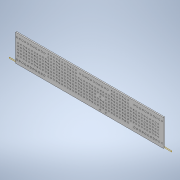
# Autodesk Inventor part: top_plate
Saved by Autodesk Inventor 2022 (Build 260153000, 153)
## iProperties
Created: 2021-07-14
Part Number: top_plate
Material: Generic
Document SubType Name: Modeling
Designer: gfellows
Density: 1 g/cm^3
Appearance: Default
Author: gfellows
Autodesk Inventor part; units mm, degrees
ref_plane "YZ Plane" through (0, 0, 0) normal (1, 0, 0) x (0, 1, 0)
ref_plane "XZ Plane" through (0, 0, 0) normal (0, 1, 0) x (-1, 0, 0)
ref_plane "XY Plane" through (0, 0, 0) normal (0, 0, 1) x (1, 0, 0)
ref_plane "Work Plane1" through (-368.7905, 0, 55) normal (0, 0, 1) x (1, 0, 0)
sketch "Sketch1" plane through (-368.7905, 0, 55) normal (0, 0, 1) x (1, 0, 0)
  line L0 (0, 0) -> (430.2, 0)
  line L1 (430.2, 0) -> (430.2, 78.35)
  line L2 (430.2, 78.35) -> (0, 78.35)
  line L3 (0, 78.35) -> (0, 0)
  circle A0 centre (262.5182, 6.225) radius 1.3525 projected
  line L4 (229.7522, 3.429) -> (229.7522, 41.021) projected
  line L5 (268.9952, 3.429) -> (229.7522, 3.429) projected
  line L6 (268.9952, 41.021) -> (268.9952, 3.429) projected
  line L7 (229.7522, 41.021) -> (268.9952, 41.021) projected
  circle A1 centre (262.5182, 6.225) radius 1.3525 projected
  circle A2 centre (246.5182, 6.225) radius 1.3525 projected
  circle A3 centre (262.5182, 38.225) radius 1.3525 projected
  circle A4 centre (246.5182, 38.225) radius 1.3525 projected
  circle A5 centre (-0.4541, 14.35) radius 1.65
  line L8 (0, 75.175) -> (0, 78.35) projected
  line L9 (0, 0) -> (430.2, 0) projected
  circle A6 centre (-0.4541, 22.35) radius 1.65
  circle A7 centre (-0.4541, 30.35) radius 1.65
  circle A8 centre (-0.4541, 38.35) radius 1.65
  circle A9 centre (-0.4541, 46.35) radius 1.65
  circle A10 centre (-0.4541, 54.35) radius 1.65
  circle A11 centre (-0.4541, 62.35) radius 1.65
  circle A12 centre (-0.4541, 70.35) radius 1.65
  circle A13 centre (7.5459, 14.35) radius 1.65
  circle A14 centre (7.5459, 22.35) radius 1.65
  circle A15 centre (7.5459, 30.35) radius 1.65
  circle A16 centre (7.5459, 38.35) radius 1.65
  circle A17 centre (7.5459, 46.35) radius 1.65
  circle A18 centre (7.5459, 54.35) radius 1.65
  circle A19 centre (7.5459, 62.35) radius 1.65
  circle A20 centre (7.5459, 70.35) radius 1.65
  circle A21 centre (15.5459, 14.35) radius 1.65
  circle A22 centre (15.5459, 22.35) radius 1.65
  circle A23 centre (15.5459, 30.35) radius 1.65
  circle A24 centre (15.5459, 38.35) radius 1.65
  circle A25 centre (15.5459, 46.35) radius 1.65
  circle A26 centre (15.5459, 54.35) radius 1.65
  circle A27 centre (15.5459, 62.35) radius 1.65
  circle A28 centre (15.5459, 70.35) radius 1.65
  circle A29 centre (23.5459, 14.35) radius 1.65
  circle A30 centre (23.5459, 22.35) radius 1.65
  circle A31 centre (23.5459, 30.35) radius 1.65
  circle A32 centre (23.5459, 38.35) radius 1.65
  circle A33 centre (23.5459, 46.35) radius 1.65
  circle A34 centre (23.5459, 54.35) radius 1.65
  circle A35 centre (23.5459, 62.35) radius 1.65
  circle A36 centre (23.5459, 70.35) radius 1.65
  circle A37 centre (31.5459, 14.35) radius 1.65
  circle A38 centre (31.5459, 22.35) radius 1.65
  circle A39 centre (31.5459, 30.35) radius 1.65
  circle A40 centre (31.5459, 38.35) radius 1.65
  circle A41 centre (31.5459, 46.35) radius 1.65
  circle A42 centre (31.5459, 54.35) radius 1.65
  circle A43 centre (31.5459, 62.35) radius 1.65
  circle A44 centre (31.5459, 70.35) radius 1.65
  circle A45 centre (39.5459, 14.35) radius 1.65
  circle A46 centre (39.5459, 22.35) radius 1.65
  circle A47 centre (39.5459, 30.35) radius 1.65
  circle A48 centre (39.5459, 38.35) radius 1.65
  circle A49 centre (39.5459, 46.35) radius 1.65
  circle A50 centre (39.5459, 54.35) radius 1.65
  circle A51 centre (39.5459, 62.35) radius 1.65
  circle A52 centre (39.5459, 70.35) radius 1.65
  circle A53 centre (47.5459, 14.35) radius 1.65
  circle A54 centre (47.5459, 22.35) radius 1.65
  circle A55 centre (47.5459, 30.35) radius 1.65
  circle A56 centre (47.5459, 38.35) radius 1.65
  circle A57 centre (47.5459, 46.35) radius 1.65
  circle A58 centre (47.5459, 54.35) radius 1.65
  circle A59 centre (47.5459, 62.35) radius 1.65
  circle A60 centre (47.5459, 70.35) radius 1.65
  circle A61 centre (55.5459, 14.35) radius 1.65
  circle A62 centre (55.5459, 22.35) radius 1.65
  circle A63 centre (55.5459, 30.35) radius 1.65
  circle A64 centre (55.5459, 38.35) radius 1.65
  circle A65 centre (55.5459, 46.35) radius 1.65
  circle A66 centre (55.5459, 54.35) radius 1.65
  circle A67 centre (55.5459, 62.35) radius 1.65
  circle A68 centre (55.5459, 70.35) radius 1.65
  circle A69 centre (63.5459, 14.35) radius 1.65
  circle A70 centre (63.5459, 22.35) radius 1.65
  circle A71 centre (63.5459, 30.35) radius 1.65
  circle A72 centre (63.5459, 38.35) radius 1.65
  circle A73 centre (63.5459, 46.35) radius 1.65
  circle A74 centre (63.5459, 54.35) radius 1.65
  circle A75 centre (63.5459, 62.35) radius 1.65
  circle A76 centre (63.5459, 70.35) radius 1.65
  circle A77 centre (71.5459, 14.35) radius 1.65
  circle A78 centre (71.5459, 22.35) radius 1.65
  circle A79 centre (71.5459, 30.35) radius 1.65
  circle A80 centre (71.5459, 38.35) radius 1.65
  circle A81 centre (71.5459, 46.35) radius 1.65
  circle A82 centre (71.5459, 54.35) radius 1.65
  circle A83 centre (71.5459, 62.35) radius 1.65
  circle A84 centre (71.5459, 70.35) radius 1.65
  circle A85 centre (79.5459, 14.35) radius 1.65
  circle A86 centre (79.5459, 22.35) radius 1.65
  circle A87 centre (79.5459, 30.35) radius 1.65
  circle A88 centre (79.5459, 38.35) radius 1.65
  circle A89 centre (79.5459, 46.35) radius 1.65
  circle A90 centre (79.5459, 54.35) radius 1.65
  circle A91 centre (79.5459, 62.35) radius 1.65
  circle A92 centre (79.5459, 70.35) radius 1.65
  circle A93 centre (87.5459, 14.35) radius 1.65
  circle A94 centre (87.5459, 22.35) radius 1.65
  circle A95 centre (87.5459, 30.35) radius 1.65
  circle A96 centre (87.5459, 38.35) radius 1.65
  circle A97 centre (87.5459, 46.35) radius 1.65
  circle A98 centre (87.5459, 54.35) radius 1.65
  circle A99 centre (87.5459, 62.35) radius 1.65
  circle A100 centre (87.5459, 70.35) radius 1.65
  circle A101 centre (95.5459, 14.35) radius 1.65
  circle A102 centre (95.5459, 22.35) radius 1.65
  circle A103 centre (95.5459, 30.35) radius 1.65
  circle A104 centre (95.5459, 38.35) radius 1.65
  circle A105 centre (95.5459, 46.35) radius 1.65
  circle A106 centre (95.5459, 54.35) radius 1.65
  circle A107 centre (95.5459, 62.35) radius 1.65
  circle A108 centre (95.5459, 70.35) radius 1.65
  circle A109 centre (103.5459, 14.35) radius 1.65
  circle A110 centre (103.5459, 22.35) radius 1.65
  circle A111 centre (103.5459, 30.35) radius 1.65
  circle A112 centre (103.5459, 38.35) radius 1.65
  circle A113 centre (103.5459, 46.35) radius 1.65
  circle A114 centre (103.5459, 54.35) radius 1.65
  circle A115 centre (103.5459, 62.35) radius 1.65
  circle A116 centre (103.5459, 70.35) radius 1.65
  circle A117 centre (111.5459, 14.35) radius 1.65
  circle A118 centre (111.5459, 22.35) radius 1.65
  circle A119 centre (111.5459, 30.35) radius 1.65
  circle A120 centre (111.5459, 38.35) radius 1.65
  circle A121 centre (111.5459, 46.35) radius 1.65
  circle A122 centre (111.5459, 54.35) radius 1.65
  circle A123 centre (111.5459, 62.35) radius 1.65
  circle A124 centre (111.5459, 70.35) radius 1.65
  circle A125 centre (119.5459, 14.35) radius 1.65
  circle A126 centre (119.5459, 22.35) radius 1.65
  circle A127 centre (119.5459, 30.35) radius 1.65
  circle A128 centre (119.5459, 38.35) radius 1.65
  circle A129 centre (119.5459, 46.35) radius 1.65
  circle A130 centre (119.5459, 54.35) radius 1.65
  circle A131 centre (119.5459, 62.35) radius 1.65
  circle A132 centre (119.5459, 70.35) radius 1.65
  circle A133 centre (127.5459, 14.35) radius 1.65
  circle A134 centre (127.5459, 22.35) radius 1.65
  circle A135 centre (127.5459, 30.35) radius 1.65
  circle A136 centre (127.5459, 38.35) radius 1.65
  circle A137 centre (127.5459, 46.35) radius 1.65
  circle A138 centre (127.5459, 54.35) radius 1.65
  circle A139 centre (127.5459, 62.35) radius 1.65
  circle A140 centre (127.5459, 70.35) radius 1.65
  circle A141 centre (135.5459, 14.35) radius 1.65
  circle A142 centre (135.5459, 22.35) radius 1.65
  circle A143 centre (135.5459, 30.35) radius 1.65
  circle A144 centre (135.5459, 38.35) radius 1.65
  circle A145 centre (135.5459, 46.35) radius 1.65
  circle A146 centre (135.5459, 54.35) radius 1.65
  circle A147 centre (135.5459, 62.35) radius 1.65
  circle A148 centre (135.5459, 70.35) radius 1.65
  circle A149 centre (143.5459, 14.35) radius 1.65
  circle A150 centre (143.5459, 22.35) radius 1.65
  circle A151 centre (143.5459, 30.35) radius 1.65
  circle A152 centre (143.5459, 38.35) radius 1.65
  circle A153 centre (143.5459, 46.35) radius 1.65
  circle A154 centre (143.5459, 54.35) radius 1.65
  circle A155 centre (143.5459, 62.35) radius 1.65
  circle A156 centre (143.5459, 70.35) radius 1.65
  circle A157 centre (151.5459, 14.35) radius 1.65
  circle A158 centre (151.5459, 22.35) radius 1.65
  circle A159 centre (151.5459, 30.35) radius 1.65
  circle A160 centre (151.5459, 38.35) radius 1.65
  circle A161 centre (151.5459, 46.35) radius 1.65
  circle A162 centre (151.5459, 54.35) radius 1.65
  circle A163 centre (151.5459, 62.35) radius 1.65
  circle A164 centre (151.5459, 70.35) radius 1.65
  circle A165 centre (159.5459, 14.35) radius 1.65
  circle A166 centre (159.5459, 22.35) radius 1.65
  circle A167 centre (159.5459, 30.35) radius 1.65
  circle A168 centre (159.5459, 38.35) radius 1.65
  circle A169 centre (159.5459, 46.35) radius 1.65
  circle A170 centre (159.5459, 54.35) radius 1.65
  circle A171 centre (159.5459, 62.35) radius 1.65
  circle A172 centre (159.5459, 70.35) radius 1.65
  circle A173 centre (167.5459, 14.35) radius 1.65
  circle A174 centre (167.5459, 22.35) radius 1.65
  circle A175 centre (167.5459, 30.35) radius 1.65
  circle A176 centre (167.5459, 38.35) radius 1.65
  circle A177 centre (167.5459, 46.35) radius 1.65
  circle A178 centre (167.5459, 54.35) radius 1.65
  circle A179 centre (167.5459, 62.35) radius 1.65
  circle A180 centre (167.5459, 70.35) radius 1.65
  circle A181 centre (175.5459, 14.35) radius 1.65
  circle A182 centre (175.5459, 22.35) radius 1.65
  circle A183 centre (175.5459, 30.35) radius 1.65
  circle A184 centre (175.5459, 38.35) radius 1.65
  circle A185 centre (175.5459, 46.35) radius 1.65
  circle A186 centre (175.5459, 54.35) radius 1.65
  circle A187 centre (175.5459, 62.35) radius 1.65
  circle A188 centre (175.5459, 70.35) radius 1.65
  circle A189 centre (183.5459, 14.35) radius 1.65
  circle A190 centre (183.5459, 22.35) radius 1.65
  circle A191 centre (183.5459, 30.35) radius 1.65
  circle A192 centre (183.5459, 38.35) radius 1.65
  circle A193 centre (183.5459, 46.35) radius 1.65
  circle A194 centre (183.5459, 54.35) radius 1.65
  circle A195 centre (183.5459, 62.35) radius 1.65
  circle A196 centre (183.5459, 70.35) radius 1.65
  circle A197 centre (191.5459, 14.35) radius 1.65
  circle A198 centre (191.5459, 22.35) radius 1.65
  circle A199 centre (191.5459, 30.35) radius 1.65
  circle A200 centre (191.5459, 38.35) radius 1.65
  circle A201 centre (191.5459, 46.35) radius 1.65
  circle A202 centre (191.5459, 54.35) radius 1.65
  circle A203 centre (191.5459, 62.35) radius 1.65
  circle A204 centre (191.5459, 70.35) radius 1.65
  circle A205 centre (199.5459, 14.35) radius 1.65
  circle A206 centre (199.5459, 22.35) radius 1.65
  circle A207 centre (199.5459, 30.35) radius 1.65
  circle A208 centre (199.5459, 38.35) radius 1.65
  circle A209 centre (199.5459, 46.35) radius 1.65
  circle A210 centre (199.5459, 54.35) radius 1.65
  circle A211 centre (199.5459, 62.35) radius 1.65
  circle A212 centre (199.5459, 70.35) radius 1.65
  circle A213 centre (207.5459, 14.35) radius 1.65
  circle A214 centre (207.5459, 22.35) radius 1.65
  circle A215 centre (207.5459, 30.35) radius 1.65
  circle A216 centre (207.5459, 38.35) radius 1.65
  circle A217 centre (207.5459, 46.35) radius 1.65
  circle A218 centre (207.5459, 54.35) radius 1.65
  circle A219 centre (207.5459, 62.35) radius 1.65
  circle A220 centre (207.5459, 70.35) radius 1.65
  circle A221 centre (215.5459, 14.35) radius 1.65
  circle A222 centre (215.5459, 22.35) radius 1.65
  circle A223 centre (215.5459, 30.35) radius 1.65
  circle A224 centre (215.5459, 38.35) radius 1.65
  circle A225 centre (215.5459, 46.35) radius 1.65
  circle A226 centre (215.5459, 54.35) radius 1.65
  circle A227 centre (215.5459, 62.35) radius 1.65
  circle A228 centre (215.5459, 70.35) radius 1.65
  circle A229 centre (223.5459, 14.35) radius 1.65
  circle A230 centre (223.5459, 22.35) radius 1.65
  circle A231 centre (223.5459, 30.35) radius 1.65
  circle A232 centre (223.5459, 38.35) radius 1.65
  circle A233 centre (223.5459, 46.35) radius 1.65
  circle A234 centre (223.5459, 54.35) radius 1.65
  circle A235 centre (223.5459, 62.35) radius 1.65
  circle A236 centre (223.5459, 70.35) radius 1.65
  circle A237 centre (231.5459, 14.35) radius 1.65
  circle A238 centre (231.5459, 22.35) radius 1.65
  circle A239 centre (231.5459, 30.35) radius 1.65
  circle A240 centre (231.5459, 38.35) radius 1.65
  circle A241 centre (231.5459, 46.35) radius 1.65
  circle A242 centre (231.5459, 54.35) radius 1.65
  circle A243 centre (231.5459, 62.35) radius 1.65
  circle A244 centre (231.5459, 70.35) radius 1.65
  circle A245 centre (239.5459, 14.35) radius 1.65
  circle A246 centre (239.5459, 22.35) radius 1.65
  circle A247 centre (239.5459, 30.35) radius 1.65
  circle A248 centre (239.5459, 38.35) radius 1.65
  circle A249 centre (239.5459, 46.35) radius 1.65
  circle A250 centre (239.5459, 54.35) radius 1.65
  circle A251 centre (239.5459, 62.35) radius 1.65
  circle A252 centre (239.5459, 70.35) radius 1.65
  circle A253 centre (247.5459, 14.35) radius 1.65
  circle A254 centre (247.5459, 22.35) radius 1.65
  circle A255 centre (247.5459, 30.35) radius 1.65
  circle A256 centre (247.5459, 38.35) radius 1.65
  circle A257 centre (247.5459, 46.35) radius 1.65
  circle A258 centre (247.5459, 54.35) radius 1.65
  circle A259 centre (247.5459, 62.35) radius 1.65
  circle A260 centre (247.5459, 70.35) radius 1.65
  circle A261 centre (255.5459, 14.35) radius 1.65
  circle A262 centre (255.5459, 22.35) radius 1.65
  circle A263 centre (255.5459, 30.35) radius 1.65
  circle A264 centre (255.5459, 38.35) radius 1.65
  circle A265 centre (255.5459, 46.35) radius 1.65
  circle A266 centre (255.5459, 54.35) radius 1.65
  circle A267 centre (255.5459, 62.35) radius 1.65
  circle A268 centre (255.5459, 70.35) radius 1.65
  circle A269 centre (263.5459, 14.35) radius 1.65
  circle A270 centre (263.5459, 22.35) radius 1.65
  circle A271 centre (263.5459, 30.35) radius 1.65
  circle A272 centre (263.5459, 38.35) radius 1.65
  circle A273 centre (263.5459, 46.35) radius 1.65
  circle A274 centre (263.5459, 54.35) radius 1.65
  circle A275 centre (263.5459, 62.35) radius 1.65
  circle A276 centre (263.5459, 70.35) radius 1.65
  circle A277 centre (271.5459, 14.35) radius 1.65
  circle A278 centre (271.5459, 22.35) radius 1.65
  circle A279 centre (271.5459, 30.35) radius 1.65
  circle A280 centre (271.5459, 38.35) radius 1.65
  circle A281 centre (271.5459, 46.35) radius 1.65
  circle A282 centre (271.5459, 54.35) radius 1.65
  circle A283 centre (271.5459, 62.35) radius 1.65
  circle A284 centre (271.5459, 70.35) radius 1.65
  circle A285 centre (279.5459, 14.35) radius 1.65
  circle A286 centre (279.5459, 22.35) radius 1.65
  circle A287 centre (279.5459, 30.35) radius 1.65
  circle A288 centre (279.5459, 38.35) radius 1.65
  circle A289 centre (279.5459, 46.35) radius 1.65
  circle A290 centre (279.5459, 54.35) radius 1.65
  circle A291 centre (279.5459, 62.35) radius 1.65
  circle A292 centre (279.5459, 70.35) radius 1.65
  circle A293 centre (287.5459, 14.35) radius 1.65
  circle A294 centre (287.5459, 22.35) radius 1.65
  circle A295 centre (287.5459, 30.35) radius 1.65
  circle A296 centre (287.5459, 38.35) radius 1.65
  circle A297 centre (287.5459, 46.35) radius 1.65
  circle A298 centre (287.5459, 54.35) radius 1.65
  circle A299 centre (287.5459, 62.35) radius 1.65
  circle A300 centre (287.5459, 70.35) radius 1.65
  circle A301 centre (295.5459, 14.35) radius 1.65
  circle A302 centre (295.5459, 22.35) radius 1.65
  circle A303 centre (295.5459, 30.35) radius 1.65
  circle A304 centre (295.5459, 38.35) radius 1.65
  circle A305 centre (295.5459, 46.35) radius 1.65
  circle A306 centre (295.5459, 54.35) radius 1.65
  circle A307 centre (295.5459, 62.35) radius 1.65
  circle A308 centre (295.5459, 70.35) radius 1.65
  circle A309 centre (303.5459, 14.35) radius 1.65
  circle A310 centre (303.5459, 22.35) radius 1.65
  circle A311 centre (303.5459, 30.35) radius 1.65
  circle A312 centre (303.5459, 38.35) radius 1.65
  circle A313 centre (303.5459, 46.35) radius 1.65
  circle A314 centre (303.5459, 54.35) radius 1.65
  circle A315 centre (303.5459, 62.35) radius 1.65
  circle A316 centre (303.5459, 70.35) radius 1.65
  circle A317 centre (311.5459, 14.35) radius 1.65
  circle A318 centre (311.5459, 22.35) radius 1.65
  circle A319 centre (311.5459, 30.35) radius 1.65
  circle A320 centre (311.5459, 38.35) radius 1.65
  circle A321 centre (311.5459, 46.35) radius 1.65
  circle A322 centre (311.5459, 54.35) radius 1.65
  circle A323 centre (311.5459, 62.35) radius 1.65
  circle A324 centre (311.5459, 70.35) radius 1.65
  circle A325 centre (319.5459, 14.35) radius 1.65
  circle A326 centre (319.5459, 22.35) radius 1.65
  circle A327 centre (319.5459, 30.35) radius 1.65
  circle A328 centre (319.5459, 38.35) radius 1.65
  circle A329 centre (319.5459, 46.35) radius 1.65
  circle A330 centre (319.5459, 54.35) radius 1.65
  circle A331 centre (319.5459, 62.35) radius 1.65
  circle A332 centre (319.5459, 70.35) radius 1.65
  circle A333 centre (327.5459, 14.35) radius 1.65
  circle A334 centre (327.5459, 22.35) radius 1.65
  circle A335 centre (327.5459, 30.35) radius 1.65
  circle A336 centre (327.5459, 38.35) radius 1.65
  circle A337 centre (327.5459, 46.35) radius 1.65
  circle A338 centre (327.5459, 54.35) radius 1.65
  circle A339 centre (327.5459, 62.35) radius 1.65
  circle A340 centre (327.5459, 70.35) radius 1.65
  circle A341 centre (335.5459, 14.35) radius 1.65
  circle A342 centre (335.5459, 22.35) radius 1.65
  circle A343 centre (335.5459, 30.35) radius 1.65
  circle A344 centre (335.5459, 38.35) radius 1.65
  circle A345 centre (335.5459, 46.35) radius 1.65
  circle A346 centre (335.5459, 54.35) radius 1.65
  circle A347 centre (335.5459, 62.35) radius 1.65
  circle A348 centre (335.5459, 70.35) radius 1.65
  circle A349 centre (343.5459, 14.35) radius 1.65
  circle A350 centre (343.5459, 22.35) radius 1.65
  circle A351 centre (343.5459, 30.35) radius 1.65
  circle A352 centre (343.5459, 38.35) radius 1.65
  circle A353 centre (343.5459, 46.35) radius 1.65
  circle A354 centre (343.5459, 54.35) radius 1.65
  circle A355 centre (343.5459, 62.35) radius 1.65
  circle A356 centre (343.5459, 70.35) radius 1.65
  circle A357 centre (351.5459, 14.35) radius 1.65
  circle A358 centre (351.5459, 22.35) radius 1.65
  circle A359 centre (351.5459, 30.35) radius 1.65
  circle A360 centre (351.5459, 38.35) radius 1.65
  circle A361 centre (351.5459, 46.35) radius 1.65
  circle A362 centre (351.5459, 54.35) radius 1.65
  circle A363 centre (351.5459, 62.35) radius 1.65
  circle A364 centre (351.5459, 70.35) radius 1.65
  circle A365 centre (359.5459, 14.35) radius 1.65
  circle A366 centre (359.5459, 22.35) radius 1.65
  circle A367 centre (359.5459, 30.35) radius 1.65
  circle A368 centre (359.5459, 38.35) radius 1.65
  circle A369 centre (359.5459, 46.35) radius 1.65
  circle A370 centre (359.5459, 54.35) radius 1.65
  circle A371 centre (359.5459, 62.35) radius 1.65
  circle A372 centre (359.5459, 70.35) radius 1.65
  circle A373 centre (367.5459, 14.35) radius 1.65
  circle A374 centre (367.5459, 22.35) radius 1.65
  circle A375 centre (367.5459, 30.35) radius 1.65
  circle A376 centre (367.5459, 38.35) radius 1.65
  circle A377 centre (367.5459, 46.35) radius 1.65
  circle A378 centre (367.5459, 54.35) radius 1.65
  circle A379 centre (367.5459, 62.35) radius 1.65
  circle A380 centre (367.5459, 70.35) radius 1.65
  circle A381 centre (375.5459, 14.35) radius 1.65
  circle A382 centre (375.5459, 22.35) radius 1.65
  circle A383 centre (375.5459, 30.35) radius 1.65
  circle A384 centre (375.5459, 38.35) radius 1.65
  circle A385 centre (375.5459, 46.35) radius 1.65
  circle A386 centre (375.5459, 54.35) radius 1.65
  circle A387 centre (375.5459, 62.35) radius 1.65
  circle A388 centre (375.5459, 70.35) radius 1.65
  circle A389 centre (383.5459, 14.35) radius 1.65
  circle A390 centre (383.5459, 22.35) radius 1.65
  circle A391 centre (383.5459, 30.35) radius 1.65
  circle A392 centre (383.5459, 38.35) radius 1.65
  circle A393 centre (383.5459, 46.35) radius 1.65
  circle A394 centre (383.5459, 54.35) radius 1.65
  circle A395 centre (383.5459, 62.35) radius 1.65
  circle A396 centre (383.5459, 70.35) radius 1.65
  circle A397 centre (391.5459, 14.35) radius 1.65
  circle A398 centre (391.5459, 22.35) radius 1.65
  circle A399 centre (391.5459, 30.35) radius 1.65
  circle A400 centre (391.5459, 38.35) radius 1.65
  circle A401 centre (391.5459, 46.35) radius 1.65
  circle A402 centre (391.5459, 54.35) radius 1.65
  circle A403 centre (391.5459, 62.35) radius 1.65
  circle A404 centre (391.5459, 70.35) radius 1.65
  circle A405 centre (399.5459, 14.35) radius 1.65
  circle A406 centre (399.5459, 22.35) radius 1.65
  circle A407 centre (399.5459, 30.35) radius 1.65
  circle A408 centre (399.5459, 38.35) radius 1.65
  circle A409 centre (399.5459, 46.35) radius 1.65
  circle A410 centre (399.5459, 54.35) radius 1.65
  circle A411 centre (399.5459, 62.35) radius 1.65
  circle A412 centre (399.5459, 70.35) radius 1.65
  circle A413 centre (407.5459, 14.35) radius 1.65
  circle A414 centre (407.5459, 22.35) radius 1.65
  circle A415 centre (407.5459, 30.35) radius 1.65
  circle A416 centre (407.5459, 38.35) radius 1.65
  circle A417 centre (407.5459, 46.35) radius 1.65
  circle A418 centre (407.5459, 54.35) radius 1.65
  circle A419 centre (407.5459, 62.35) radius 1.65
  circle A420 centre (407.5459, 70.35) radius 1.65
  circle A421 centre (415.5459, 14.35) radius 1.65
  circle A422 centre (415.5459, 22.35) radius 1.65
  circle A423 centre (415.5459, 30.35) radius 1.65
  circle A424 centre (415.5459, 38.35) radius 1.65
  circle A425 centre (415.5459, 46.35) radius 1.65
  circle A426 centre (415.5459, 54.35) radius 1.65
  circle A427 centre (415.5459, 62.35) radius 1.65
  circle A428 centre (415.5459, 70.35) radius 1.65
  line L10 (0, 78.35) -> (430.2, 78.35) projected
  line L11 (117.0709, 342.35) -> (106.0209, 342.35) projected
  line L12 (117.0709, 342.35) -> (117.0709, 78.35)
  line L13 (117.0709, 210.35) -> (0, 210.35)
  line L14 (0, 75.175) -> (0, 63.175) projected
  line L15 (280, 63.175) -> (0, 63.175) projected
  line L16 (280, 75.175) -> (280, 63.175) projected
  line L17 (280, 75.175) -> (0, 75.175) projected
  circle A429 centre (4, 67.175) radius 2 projected
  circle A430 centre (12, 67.175) radius 2 projected
  circle A431 centre (20, 67.175) radius 2 projected
  circle A432 centre (28, 67.175) radius 2 projected
  circle A433 centre (36, 67.175) radius 2 projected
  circle A434 centre (44, 67.175) radius 2 projected
  circle A435 centre (52, 67.175) radius 2 projected
  circle A436 centre (60, 67.175) radius 2 projected
  circle A437 centre (68, 67.175) radius 2 projected
  circle A438 centre (76, 67.175) radius 2 projected
  circle A439 centre (84, 67.175) radius 2 projected
  circle A440 centre (92, 67.175) radius 2 projected
  circle A441 centre (100, 67.175) radius 2 projected
  circle A442 centre (108, 67.175) radius 2 projected
  circle A443 centre (116, 67.175) radius 2 projected
  circle A444 centre (124, 67.175) radius 2 projected
  circle A445 centre (132, 67.175) radius 2 projected
  circle A446 centre (140, 67.175) radius 2 projected
  circle A447 centre (148, 67.175) radius 2 projected
  circle A448 centre (156, 67.175) radius 2 projected
  circle A449 centre (164, 67.175) radius 2 projected
  circle A450 centre (172, 67.175) radius 2 projected
  circle A451 centre (180, 67.175) radius 2 projected
  circle A452 centre (188, 67.175) radius 2 projected
  circle A453 centre (196, 67.175) radius 2 projected
  circle A454 centre (204, 67.175) radius 2 projected
  circle A455 centre (212, 67.175) radius 2 projected
  circle A456 centre (220, 67.175) radius 2 projected
  circle A457 centre (228, 67.175) radius 2 projected
  circle A458 centre (236, 67.175) radius 2 projected
  circle A459 centre (244, 67.175) radius 2 projected
  circle A460 centre (252, 67.175) radius 2 projected
  circle A461 centre (260, 67.175) radius 2 projected
  circle A462 centre (268, 67.175) radius 2 projected
  circle A463 centre (276, 67.175) radius 2 projected
  line L18 (342.2, 75.175) -> (342.2, 63.175) projected
  line L19 (430.2, 63.175) -> (342.2, 63.175) projected
  line L20 (430.2, 75.175) -> (430.2, 63.175) projected
  line L21 (430.2, 75.175) -> (342.2, 75.175) projected
  circle A464 centre (346.2, 67.175) radius 2 projected
  circle A465 centre (354.2, 67.175) radius 2 projected
  circle A466 centre (362.2, 67.175) radius 2 projected
  circle A467 centre (370.2, 67.175) radius 2 projected
  circle A468 centre (378.2, 67.175) radius 2 projected
  circle A469 centre (386.2, 67.175) radius 2 projected
  circle A470 centre (394.2, 67.175) radius 2 projected
  circle A471 centre (402.2, 67.175) radius 2 projected
  circle A472 centre (410.2, 67.175) radius 2 projected
  circle A473 centre (418.2, 67.175) radius 2 projected
  circle A474 centre (426.2, 67.175) radius 2 projected
  line L22 (342.2, 3.175) -> (342.2, 15.175) projected
  line L23 (430.2, 3.175) -> (342.2, 3.175) projected
  line L24 (430.2, 3.175) -> (430.2, 15.175) projected
  line L25 (430.2, 15.175) -> (342.2, 15.175) projected
  circle A475 centre (362.2, 11.175) radius 2 projected
  circle A476 centre (370.2, 11.175) radius 2 projected
  circle A477 centre (378.2, 11.175) radius 2 projected
  circle A478 centre (386.2, 11.175) radius 2 projected
  circle A479 centre (394.2, 11.175) radius 2 projected
  circle A480 centre (402.2, 11.175) radius 2 projected
  circle A481 centre (410.2, 11.175) radius 2 projected
  circle A482 centre (418.2, 11.175) radius 2 projected
  circle A483 centre (426.2, 11.175) radius 2 projected
  circle A484 centre (354.2, 11.175) radius 2 projected
  circle A485 centre (346.2, 11.175) radius 2 projected
  line L26 (0, 3.175) -> (0, 15.175) projected
  line L27 (88, 3.175) -> (0, 3.175) projected
  line L28 (88, 3.175) -> (88, 15.175) projected
  line L29 (88, 15.175) -> (0, 15.175) projected
  circle A486 centre (20, 11.175) radius 2 projected
  circle A487 centre (28, 11.175) radius 2 projected
  circle A488 centre (36, 11.175) radius 2 projected
  circle A489 centre (44, 11.175) radius 2 projected
  circle A490 centre (52, 11.175) radius 2 projected
  circle A491 centre (60, 11.175) radius 2 projected
  circle A492 centre (68, 11.175) radius 2 projected
  circle A493 centre (76, 11.175) radius 2 projected
  circle A494 centre (84, 11.175) radius 2 projected
  circle A495 centre (12, 11.175) radius 2 projected
  circle A496 centre (4, 11.175) radius 2 projected
  line L30 (115.5459, 78.35) -> (115.5459, 342.35) projected
  line L31 (107.5459, 78.35) -> (107.5459, 342.35) projected
  line L32 (115.5459, 78.35) -> (107.5459, 78.35)
  line L33 (111.5459, 78.35) -> (111.5459, 57.9854) construction
  point P0 (368.7905, 0)
  point P1 (118.0382, 342.35)
  dimension "d7" = 3.3
  dimension "d10" = 8
  dimension "d13" = 8
  dimension "d16" = 140
  constraints: 424 centre point, 16 end point, 4 horizontal, 2 midpoint, 2 parallel, 2 perpendicular, 2 point on line, 2 vertical, 849 other
  measures "d7" diameter of A5
  measures "d10" distance of A5.centre A6.centre
  measures "d13" distance of A5.centre A13.centre
  measures "d16" distance from line of L13 A12.centre
extrude "Extrusion1" add sketch "Sketch1" along normal blind 3.175 contours L3 L27 L28 A93 L29 A85 A77 A69 A61 A53 A45 A37 A29 A21 A13 A5 A6 A7 A8 A9 A10 A11 L15 A19 A27 A35 A43 A51 A59 A67 A75 A83 A91 A99 A107 A115 A123 A131 A139 A147 A155 A163 A171 A179 A187 A195 A203 A211 A219 A227 A235 A243 A251 A259 A267 A275 A283 A291 L16 A292 L17 L2 L1 L21 L18 A356 A355 L19 A363 A371 A379 A387 A395 A403 A411 A419 A427 L25 A421 A413 A405 A397 A389 A381 A373 A365 A357 A349 L22 L23 L0 | L3 A5 L29 A13 A21 A29 A37 A45 A53 A61 A69 A77 A85 A93 L28 L27 | L23 L22 A349 L25 A357 A365 A373 A381 A389 A397 A405 A413 A421 L1 | L3 L29 A5 | L3 A5 L29 | L28 L29 A93 | A93 L29 L28 | L19 A427 A419 A411 A403 A395 A387 A379 A371 A363 A355 L18 A356 L21 L1 | L25 A421 | A421 L25 | L22 L25 A349 | A349 L25 L22 | L3 A6 | L19 A427 | A427 L19 | L29 A13 | A13 L29 | L29 A85 | A85 L29 | L25 A413 | A413 L25 | L25 A357 | A357 L25 | L3 A7 | L18 A356 | A356 L18 | L19 A419 | A419 L19 | L29 A21 | A21 L29 | L29 A77 | A77 L29 | L25 A405 | A405 L25 | L25 A365 | A365 L25 | L3 A8 | L18 L19 A355 | A355 L19 L18 | L19 A411 | A411 L19 | L29 A29 | A29 L29 | L29 A69 | A69 L29 | L25 A397 | A397 L25 | L25 A373 | A373 L25 | L3 A9 | L17 L16 A292 A291 L15 A283 A275 A267 A259 A251 A243 A235 A227 A219 A211 A203 A195 A187 A179 A171 A163 A155 A147 A139 A131 A123 A115 A107 A99 A91 A83 A75 A67 A59 A51 A43 A35 A27 A19 A11 L3 A12 | L19 A363 | A363 L19 | L19 A403 | A403 L19 | L29 A37 | A37 L29 | L29 A61 | A61 L29 | A12 L3 | L25 A389 | A389 L25 | L25 A381 | A381 L25 | L3 A10 | L19 A371 | A371 L19 | L19 A395 | A395 L19 | L29 A45 | A45 L29 | L29 A53 | A53 L29 | A11 L15 L3 | L3 L15 A11 | L19 A379 | A379 L19 | L19 A387 | A387 L19 | L15 A19 | A19 L15 | L15 A283 | A283 L15 | L15 A27 | A27 L15 | L15 A275 | A275 L15 | L15 A35 | A35 L15 | L15 A267 | A267 L15 | L15 A43 | A43 L15 | L15 A259 | A259 L15 | L15 A51 | A51 L15 | L15 A251 | A251 L15 | L15 A59 | A59 L15 | L15 A243 | A243 L15 | L15 A67 | A67 L15 | L15 A235 | A235 L15 | L15 A75 | A75 L15 | L15 A227 | A227 L15 | L15 A83 | A83 L15 | L15 A219 | A219 L15 | L15 A91 | A91 L15 | L15 A211 | A211 L15 | L15 A99 | A99 L15 | L15 A203 | A203 L15 | L15 A195 | A195 L15 | L4 L7 L6 L5 | A3 A272 | A4 A256 | A20 | A28 | A36 | A44 | A52 | A60 | A68 | A76 | A84 | A92 | A100 | A196 | A204 | A212 | A220 | A228 | A236 | A244 | A248 | A252 | A260 | A264 | A268 | A276 | A284 | A341 | A347 | A348 | A364 | A372 | A380 | A388 | A396 | A404 | A412 | A420 | A428 | A440 | A441 | A442 | A443 | A444 | A445 | A446 | A447 | A448 | A449 | A450 | A451 | A463 picked at (0.3973, 21.9744) picked at (0.3973, 29.9744) picked at (0.6049, 38.2325) picked at (0.6049, 46.2325) picked at (0.5068, 70.6811) picked at (0.6049, 54.2325) picked at (264.7275, 38.5379) picked at (248.7275, 38.5379)
body "Solid1"
